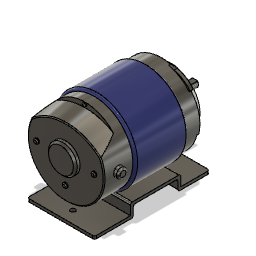
motor (Autodesk Fusion 360 design; units mm, degrees)
Autodesk Fusion 360 part; units mm, degrees
note: some values were not read from the file. Chosen so that the rebuilt part matches the saved one: which face or edge a step refers to. Set by a fixed rule: which sketch regions a step uses.
sketch "Sketch1" plane through (0, 0, 0) normal (0, 0, 1) x (1, 0, 0)
  circle A0 centre (0, 0) radius 42.5
  dimension "d1" = 85
  constraint coincident A0.centre origin
  measures "d1" diameter of A0
extrude "Extrude1" add sketch "Sketch1" along normal mid plane 240
ref_plane "WorkPlane1" through (0, 0, 85) normal (0, 0, 1) x (1, 0, 0)
ref_plane "WorkPlane2" through (0, 0, 95) normal (0, 0, 1) x (1, 0, 0)
sketch "Sketch2" plane through (0, 0, 85) normal (0, 0, 1) x (1, 0, 0)
sketch "Sketch3" plane through (0, 0, 95) normal (0, 0, 1) x (1, 0, 0)
ref_plane "WorkPlane3" through (0, 0, 95) normal (0, 0, 1) x (1, 0, 0)
sketch "Sketch4" plane through (0, 0, 95) normal (0, 0, 1) x (1, 0, 0)
sketch "Sketch5" plane through (0, 0, 95) normal (0, 0, 1) x (1, 0, 0)
sketch "Sketch9" plane through (0, 0, 120) normal (0, 0, 1) x (1, 0, 0)
  circle A0 centre (0, 0) radius 42.5
  arc A1 (41.2919, 10.0612) -> (-41.3271, 9.9158) centre (0.0399, -22.6432) ccw
  arc A2 (41.2919, 10.0612) -> (-41.3271, 9.9158) centre (-0.0158, 8.9798) ccw
  constraint coincident A0 A1.start
  constraint coincident A0 A1.end
extrude "Extrude2" cut sketch "Sketch9" against normal blind 25 contours A0 A1 | A0 A2 picked at (-0.06, 34.0821)
chamfer "Chamfer1" distance 25 distance2 5 1 edges at (-0.0528, 29.9999, 95) measured on face at (15.5458, 27.6646, 103.3333)
sketch "Sketch10" plane through (0, 0, 120) normal (0, 0, 1) x (1, 0, 0)
  arc A0 (41.2919, 10.0612) -> (-41.3271, 9.9158) centre (0.0399, -22.6432) ccw
  arc A1 (-41.3271, 9.9158) -> (41.2919, 10.0612) centre (0, 0) ccw
  circle A2 centre (0, 0) radius 15
  circle A3 centre (0, 0) radius 42.5
  dimension "d12" = 30
  constraint concentric A1 A2
  constraint concentric A2 A3
  measures "d12" diameter of A2
extrude "Extrude3" cut sketch "Sketch10" against normal blind 5
sketch "Sketch11" plane through (0, 0, 0) normal (1, 0, 0) x (0, 0, -1)
sketch "Sketch12" plane through (0, 0, 0) normal (0, 1, 0) x (1, 0, 0)
  line L0 (0, -120) -> (0, 0)
  constraint coincident L0.end origin
sketch "Sketch13" plane through (0, 0, 0) normal (0, 0, 1) x (1, 0, 0)
  circle A0 centre (0, 0) radius 63.2456
  constraint coincident A0.centre origin
extrude "Extrude4" cut sketch "Sketch13" against normal blind 160
sketch "Sketch14" plane through (0, 0, 0) normal (0, 1, 0) x (1, 0, 0)
sketch "Sketch15" plane through (0, 0, 85) normal (0, 0, 1) x (1, 0, 0)
  circle A0 centre (0, 0) radius 40
  circle A1 centre (0, 0) radius 42.5
  circle A2 centre (0, 0) radius 42.5
  arc A3 (36.2233, 22.2288) -> (-36.3014, 22.1011) centre (0, 0) ccw
  dimension "d17" = 80
  constraint coincident A0.centre A1.centre
  constraint concentric A0 A1
  measures "d17" diameter of A0
extrude "Extrude5" cut sketch "Sketch15" along normal blind 90
fillet "Fillet1" radius 2.5 1 edges at (-39.6239, 15.3687, 85)
ref_plane "WorkPlane4" through (0, 0, 30) normal (0, 0, -1) x (-1, 0, 0)
sketch "Sketch16" plane through (0, 0, 30) normal (0, 0, -1) x (1, 0, 0)
  circle A0 centre (0, 0) radius 40
  circle A1 centre (0, 0) radius 42.5
  circle A2 centre (0, 0) radius 42.5
  dimension "d22" = 80
  constraint coincident A0.centre A1.centre
  constraint concentric A0 A1
  measures "d22" diameter of A0
extrude "Extrude6" cut sketch "Sketch16" along normal blind 70
fillet "Fillet2" radius 2 1 edges at (-39.6239, -15.3687, 30)
sketch "Sketch17" plane through (0, 0, 0) normal (0, 0, -1) x (-1, 0, 0)
  circle A0 centre (0, 0) radius 40
  circle A1 centre (0, 0) radius 15
  circle A2 centre (0, 0) radius 15
  dimension "d26" = 30
  constraint concentric A0 A1
  measures "d26" diameter of A1
extrude "Extrude7" cut sketch "Sketch17" against normal blind 5
chamfer "Chamfer2" distance 10 angle 45 1 edges at (-37.2931, -14.4646, 5)
sketch "Sketch18" plane through (0, 0, 0) normal (1, 0, 0) x (0, 0, -1)
sketch "Sketch19" plane through (0, 0, 0) normal (1, 0, 0) x (0, 0, -1)
  line L0 (-115, 15) -> (-115, -15)
  line L1 (-120, 15) -> (-120, -15)
  line L2 (0, -15) -> (0, 15)
  line L3 (-7, 0) -> (-85, 0)
  line L4 (-85, -40) -> (-85, 40)
  line L5 (-15, -40) -> (-15, 40)
  line L6 (-85, 37.8444) -> (-16.9916, 37.8444)
  line L7 (-16.9916, 37.8444) -> (-7, 28)
  line L8 (-7, 28) -> (-7, 0)
  line L9 (-7, 0) -> (-85, 0)
  point P0 (-120, 0)
  constraint coincident L3.end L9.end
  constraint coincident L4 L6.start
  constraint perpendicular L5 L6
  constraint parallel L5 L8
revolve "Revolve1" cut sketch "Sketch19" angle 360 about axis through (0, 0, 7) along (0, 0, 1) contours L3 L4 L5 L6 L7 L9
sketch "Sketch20" plane through (0, 0, 0) normal (0, 0, 1) x (1, 0, 0)
  circle A0 centre (0, 0) radius 4
  constraint coincident A0.centre origin
extrude "Extrude8" cut sketch "Sketch20" along normal blind 57
sketch "Sketch21" plane through (0, 0, 16.9916) normal (0, 0, 1) x (1, 0, 0)
  circle A0 centre (0, 0) radius 37.8444
  circle A1 centre (0, 0) radius 29.3451
  circle A2 centre (0, 0) radius 40
  line L0 (30.8065, 25.5139) -> (23.0524, 18.1583)
  line L1 (6.3754, 28.6442) -> (9.3426, 38.8936)
  arc A3 (30.8065, 25.5139) -> (9.3426, 38.8936) centre (0, 0) ccw
  arc A4 (23.0524, 18.1583) -> (6.3754, 28.6442) centre (-0.1137, -0.1809) ccw
  constraint coincident A2 L0.start
  constraint coincident A1 L0.end
  constraint coincident A1 L1.start
  constraint coincident A2 L1.end
extrude "Extrude10" cut sketch "Sketch21" against normal blind 29 contours A0 A1 L0 L1 | A0 A2 L0 L1 A3 picked at (25.1585, 24.2584)
revolve "Revolve2" cut sketch "Sketch19" angle 360 about axis through (0, 0, 7) along (0, 0, 1)
sketch "Sketch22" plane through (0, 0, 16.9916) normal (0, 0, 1) x (1, 0, 0)
pattern_circular "C-Pattern1" count 4 over 360 about axis through (0, 0, 0) along (0, 0, 1) of "Extrude10"
sketch "Sketch23" plane through (0, 0, 0) normal (1, 0, 0) x (0, 0, -1)
  line L0 (-7, 0) -> (-85, 0)
  line L1 (-16.9916, 28.6442) -> (-16.9916, 18.1583)
  line L2 (-18.3961, 4) -> (-18.3961, 20)
  line L3 (-30, 40) -> (-30, -40)
  line L4 (-30, 40.5) -> (-30, -40.5)
  line L5 (-18.3961, 20) -> (-30, 20)
  line L6 (-30, 27.8576) -> (-65, 27.8576)
  line L7 (-65, 27.8576) -> (-65, 0)
  line L8 (-18.3961, 0) -> (0, 0)
  line L9 (0, 2) -> (0, 4)
  line L10 (0, 0) -> (20, 0)
  line L11 (20, 0) -> (20, 4)
  line L12 (20, 4) -> (-18.3961, 4)
  dimension "d40" = 4
  dimension "d41" = 90
  dimension "d42" = 4
  constraint coincident L0 L8.start
  constraint parallel L1 L2
  constraint coincident L3 L5.end
  constraint coincident L4 L6.start
  constraint perpendicular L4 L6
  constraint coincident L0 L7.end
  constraint perpendicular L0 L7
  constraint coincident L8.end L10.start
  constraint vertical L9
  constraint perpendicular L9 L10
  constraint perpendicular L2 L12
  measures "d40" distance of L8.end L9.end
  measures "d41" angle of L10 L11
  measures "d42" distance of L10.end L11.end
revolve "Revolve3" add sketch "Sketch23" angle 360 about axis through (0, 0, 7) along (0, 0, 1)
fillet "Fillet3" radius 2.5 1 edges at (-18.6465, 7.2323, 18.3961)
sketch "Sketch24" plane through (0, 0, 0) normal (1, 0, 0) x (0, 0, -1)
sketch "Sketch25" plane through (0, 0, -20) normal (0, 0, -1) x (-1, 0, 0)
  circle A0 centre (0, 0) radius 4
  line L0 (-5, 3) -> (5, 3)
  line L1 (5, 3) -> (5, 5.5606)
  line L2 (5, 5.5606) -> (-5, 5.5606)
  line L3 (-5, 5.5606) -> (-5, 3)
  constraint horizontal L0
  constraint perpendicular L0 L1
  constraint perpendicular L1 L2
  constraint perpendicular L0 L3
extrude "Extrude11" cut sketch "Sketch25" against normal blind 12 contours A0 L0 picked at (-0.3801, 3.278)
fillet "Fillet4" radius 0.5 1 edges at (0, -4, -20)
sketch "Sketch26" plane through (0, 0, 0) normal (0, 0, -1) x (-1, 0, 0)
  circle A0 centre (0, 0) radius 4
  circle A1 centre (0, 0) radius 15
  line L0 (-10, 2) -> (-11.7321, 1)
  line L1 (-11.7321, -1) -> (-10, -2)
  line L2 (-10, -2) -> (-8.2679, -1)
  line L3 (-8.2679, -1) -> (-8.2679, 1)
  line L4 (-8.2679, 1) -> (-10, 2)
  line L5 (-11.7321, 1) -> (-11.7321, -1)
  line L6 (10, 2) -> (8.2679, 1)
  line L7 (8.2679, 1) -> (8.2679, -1)
  line L8 (8.2679, -1) -> (10, -2)
  line L9 (10, -2) -> (11.7321, -1)
  line L10 (11.7321, -1) -> (11.7321, 1)
  line L11 (11.7321, 1) -> (10, 2)
  circle A2 centre (10, 0) radius 1.2632
  circle A3 centre (-10, 0) radius 1.2239
  constraint parallel L0 L2
  constraint vertical L3
  constraint parallel L1 L4
  constraint parallel L5 L7
  constraint parallel L6 L9
sketch "Sketch27" plane through (0, 0, 0) normal (0, 0, -1) x (-1, 0, 0)
  line L0 (16, 2.5) -> (16, -2.5)
  line L1 (-16, -2.5) -> (-16, 2.5)
  arc A0 (-10, -2.5) -> (-10, 2.5) centre (-10, 0) ccw
  arc A1 (10, 2.5) -> (10, -2.5) centre (10, 0) ccw
  line L2 (-16, 2.5) -> (-10, 2.5)
  line L3 (10, 2.5) -> (16, 2.5)
  line L4 (16, -2.5) -> (10, -2.5)
  line L5 (-10, -2.5) -> (-16, -2.5)
  constraint horizontal L2
  constraint perpendicular L0 L2
  constraint perpendicular L0 L4
  constraint perpendicular L1 L2
  constraint tangent A0 L4
  constraint tangent A0 L2
  constraint coincident A0.start L4
  constraint tangent A1 L4
  constraint tangent A1 L2
  constraint coincident A1.start L2
  constraint collinear L2 L3
  constraint collinear L4 L5
extrude "Extrude12" cut sketch "Sketch27" against normal blind 2
extrude "Extrude13" add sketch "Sketch26" along normal blind 1 and the other way blind 2 contours L0 L1 L2 L3 L4 L5 | L6 L7 L8 L9 L10 L11
sketch "Sketch28" plane through (0, 0, 0) normal (0, 0, -1) x (-1, 0, 0)
  line L0 (14.7902, -2.5) -> (10, -2.5)
  arc A0 (10, 2.5) -> (10, -2.5) centre (10, 0) ccw
  line L1 (10, 2.5) -> (14.7902, 2.5)
  arc A1 (14.7902, 2.5) -> (-14.7902, 2.5) centre (0, 0) ccw
  line L2 (-14.7902, 2.5) -> (-10, 2.5)
  arc A2 (-10, -2.5) -> (-10, 2.5) centre (-10, 0) ccw
  line L3 (-10, -2.5) -> (-14.7902, -2.5)
  arc A3 (-14.7902, -2.5) -> (14.7902, -2.5) centre (0, 0) ccw
  circle A4 centre (0, 0) radius 4
  circle A5 centre (0, 0) radius 4
  circle A6 centre (0, 0) radius 5
  line L4 (0, -15) -> (0, 15)
  line L5 (0, -40) -> (0, 40)
  constraint coincident A1.centre A3.centre
extrude "Extrude14" cut sketch "Sketch28" against normal blind 2 contours A4 A5 A6 L4 L5 | A4 A5 A6 L4 L5
sketch "Sketch29" plane through (0, 0, 95) normal (0, 0, 1) x (1, 0, 0)
  arc A0 (29.72, 26.7717) -> (-29.814, 26.6669) centre (0, 0) ccw
  arc A1 (29.72, 26.7717) -> (-29.814, 26.6669) centre (0.0399, -22.6432) ccw
  circle A2 centre (0, 37.8444) radius 1.8444
  line L0 (0, -40) -> (0, 40)
  line L1 (0, 37.8444) -> (0, 28)
  point P0 (0, 37.8444)
  constraint coincident P0 A2.centre
extrude "Extrude15" add sketch "Sketch29" along normal blind 2 contours A2 L0 L1 | A2 L0 L1
fillet "Fillet5" radius 1 1 edges at (-1.7196, 37.1774, 97)
sketch "Sketch30" plane through (0, 0, 115) normal (0, 0, 1) x (1, 0, 0)
  arc A0 (-36.2889, 16.8259) -> (36.2295, 16.9536) centre (0, 0) ccw
  arc A1 (36.2295, 16.9536) -> (-36.2889, 16.8259) centre (0.0399, -22.6432) ccw
  circle A2 centre (0, 0) radius 15
  circle A3 centre (30, 0) radius 2.5
  circle A4 centre (-30, 0) radius 2.5
  arc A5 (-29.2745, 6.5579) -> (-23.5295, -18.6108) centre (0, 0) ccw
  circle A6 centre (0, -25) radius 2.5
  line L0 (0, -40) -> (0, 40)
  dimension "d59" = 5
  dimension "d60" = 5
  dimension "d61" = 5
  constraint coincident A4.centre A5
  constraint coincident A6.centre L0
  measures "d59" diameter of A3
  measures "d60" diameter of A4
  measures "d61" diameter of A6
extrude "Extrude16" add sketch "Sketch30" along normal blind 2 contours A6 L0 | A6 L0 | A3 | A4 A5 | A4 A5
chamfer "Chamfer3" distance 1 angle 45 3 edges at (-32.3308, -0.904, 117) (27.6692, -0.904, 117) (-2.3308, -25.904, 117)
chamfer "Chamfer4" distance 2 angle 45 1 edges at (-13.9849, -5.4242, 120)
sketch "Sketch31" plane through (0, 0, 0) normal (0, 0, 1) x (1, 0, 0)
sketch "Sketch32" plane through (0, 0, 0) normal (0, 0, -1) x (-1, 0, 0)
  circle A0 centre (0, 0) radius 5
  line L0 (14.7902, -2.5) -> (10, -2.5)
  arc A1 (10, 2.5) -> (10, -2.5) centre (10, 0) ccw
  line L1 (10, 2.5) -> (14.7902, 2.5)
  arc A2 (14.7902, 2.5) -> (-14.7902, 2.5) centre (0, 0) ccw
  line L2 (-14.7902, 2.5) -> (-10, 2.5)
  arc A3 (-10, -2.5) -> (-10, 2.5) centre (-10, 0) ccw
  line L3 (-10, -2.5) -> (-14.7902, -2.5)
  arc A4 (-14.7902, -2.5) -> (14.7902, -2.5) centre (0, 0) ccw
  line L4 (0, -40) -> (0, 40)
  line L5 (0, 0) -> (0, -75)
  line L6 (0, -75) -> (45, -75)
  line L7 (45, -75) -> (45, -40)
  circle A5 centre (0, 0) radius 42.5
  line L8 (0, -75) -> (-45, -75)
  line L9 (-45, -75) -> (-45, -40)
  arc A6 (-14.3614, -40) -> (14.3614, -40) centre (0, 0) ccw
  line L10 (-45, -40) -> (-14.3614, -40)
  line L11 (14.3614, -40) -> (45, -40)
  constraint coincident A0.centre A2.centre
  constraint parallel L4 L5
  constraint perpendicular L5 L6
  constraint perpendicular L6 L7
  constraint perpendicular L5 L8
  constraint perpendicular L8 L9
  constraint perpendicular L7 L10
  constraint coincident A6.end L10
  constraint coincident A5 A6.end
  constraint coincident A5 A6.start
  constraint collinear L10 L11
extrude "Extrude17" add sketch "Sketch32" against normal blind 120 contours L5 L6 L7 A5 A6 L11 | L5 A5 L8 L9 A6 L10
sketch "Sketch33" plane through (-45, 0, 0) normal (-1, 0, 0) x (0, 0, 1)
  line L0 (0, -40) -> (0, -75)
  line L1 (0, -75) -> (120, -75)
  line L2 (120, -75) -> (120, -40)
  line L3 (120, -40) -> (0, -40)
  line L4 (30, -40) -> (-10, -40)
  line L5 (-10, -40) -> (-10, -72)
  line L6 (-10, -72) -> (30, -72)
  line L7 (30, -72) -> (30, -40)
  line L8 (82.5, -40) -> (82.5, -72)
  line L9 (82.5, -72) -> (127.3639, -72)
  line L10 (127.3639, -72) -> (125, -40)
  line L11 (125, -40) -> (82.5, -40)
  point P0 (82.5, -40)
  point P1 (82.5, -40)
  dimension "d70" = 90
  dimension "d71" = 32
  constraint coincident L3 L4.start
  constraint perpendicular L0 L4
  constraint perpendicular L0 L6
  constraint perpendicular L4 L7
  constraint coincident P1 P0
  constraint perpendicular L3 L8
  constraint perpendicular L2 L9
  constraint perpendicular L8 L11
  measures "d70" angle of L4 L5
  measures "d71" distance of L4.end L5.end
extrude "Extrude18" cut sketch "Sketch33" against normal blind 320 contours L0 L3 L4 L6 L7 | L0 L4 L5 L6 | L2 L3 L8 L9 L11 | L2 L9 L10 L11
sketch "Sketch34" plane through (-45, 0, 0) normal (-1, 0, 0) x (0, 0, 1)
  line L0 (30, -72) -> (0, -72)
  line L1 (0, -72) -> (0, -75)
  line L2 (0, -75) -> (120, -75)
  line L3 (120, -75) -> (120, -72)
  line L4 (120, -72) -> (82.5, -72)
  line L5 (82.5, -40) -> (30, -40)
  line L6 (33, -43) -> (33, -72)
  line L7 (79.5, -72) -> (79.5, -43)
  line L8 (79.5, -43) -> (33, -43)
  line L9 (33, -72) -> (33, -81.992)
  line L10 (79.5, -72) -> (79.5, -81.8501)
  line L11 (79.5, -81.8501) -> (35.0278, -81.992)
  line L12 (35.0278, -81.992) -> (33, -81.992)
  constraint parallel L5 L8
  constraint perpendicular L2 L9
  constraint perpendicular L2 L10
  constraint perpendicular L9 L12
extrude "Extrude19" cut sketch "Sketch34" against normal blind 120
sketch "Sketch35" plane through (0, 0, 30) normal (0, 0, -1) x (-1, 0, 0)
  arc A0 (-14.3614, -40) -> (14.3614, -40) centre (0, 0) ccw
  line L0 (-14.3614, -40) -> (-45, -40)
  line L1 (-45, -40) -> (-45, -72)
  line L2 (-45, -72) -> (45, -72)
  line L3 (45, -72) -> (45, -40)
  line L4 (45, -40) -> (14.3614, -40)
  line L5 (-35, -40) -> (-35, -87.1803)
  line L6 (-35, -87.1803) -> (-60.0488, -77.3043)
  line L7 (-60.0488, -77.3043) -> (-58.0333, -25.1025)
  line L8 (-58.0333, -25.1025) -> (-35, -31.9553)
  line L9 (-35, -31.9553) -> (-35, -40)
  line L10 (35, -85) -> (35, -31.9553)
  line L11 (35, -31.9553) -> (53.2229, -31.9553)
  line L12 (53.2229, -31.9553) -> (50, -85)
  line L13 (50, -85) -> (35, -85)
  constraint coincident L0 L5.start
  constraint perpendicular L2 L5
  constraint perpendicular L0 L9
  constraint perpendicular L2 L10
  constraint perpendicular L10 L11
  constraint perpendicular L10 L13
extrude "Extrude20" cut sketch "Sketch35" along normal mid plane 270 contours L0 L1 L2 L5 | L0 L1 L2 L5 L6 L7 L8 L9 | L2 L3 L4 L10 L11 L12 L13 | L2 L3 L4 L10
fillet "Fillet6" radius 2 1 edges at (0, -72, 30)
fillet "Fillet7" radius 2 5 edges at (24.6807, -40, 30) (-24.6807, -40, 30) (-24.6807, -40, 82.5) (24.6807, -40, 82.5) (0, -72, 82.5)
fillet "Fillet8" radius 2 4 edges at (0, -75, 33) (0, -43, 33) (0, -43, 79.5) (0, -75, 79.5)
sketch "Sketch36" plane through (0, -72, 0) normal (0, 1, 0) x (-1, 0, 0)
  line L0 (35, 28) -> (-35, 28)
  line L1 (-35, 28) -> (-35, 0)
  line L2 (-35, 0) -> (35, 0)
  line L3 (35, 0) -> (35, 28)
  line L4 (0, 16.9916) -> (0, 7)
  line L5 (0, 11.9958) -> (0, 96.9958)
  line L6 (-25, 14.9958) -> (25, 14.9958)
  line L7 (25, 14.9958) -> (25, 8.9958)
  line L8 (25, 8.9958) -> (-25, 8.9958)
  line L9 (-25, 8.9958) -> (-25, 14.9958)
  line L10 (-25, 14.9958) -> (25, 8.9958) construction
  line L11 (25, 14.9958) -> (-25, 8.9958) construction
  line L12 (-25, 99.9958) -> (25, 99.9958)
  line L13 (25, 99.9958) -> (25, 93.9958)
  line L14 (25, 93.9958) -> (-25, 93.9958)
  line L15 (-25, 93.9958) -> (-25, 99.9958)
  line L16 (-25, 99.9958) -> (25, 93.9958) construction
  line L17 (25, 99.9958) -> (-25, 93.9958) construction
  point P0 (0, 11.9958)
  point P1 (0, 96.9958)
  dimension "d82" = 85
  dimension "d83" = 50
  dimension "d84" = 6
  dimension "d85" = 50
  dimension "d86" = 6
  constraint midpoint L4 P0
  constraint perpendicular L0 L5
  constraint perpendicular L6 L7
  constraint parallel L6 L8
  constraint parallel L7 L9
  constraint horizontal L6
  constraint coincident L10 P0
  constraint coincident L11 P0
  constraint coincident P0 L5.start
  constraint perpendicular L12 L13
  constraint parallel L12 L14
  constraint parallel L13 L15
  constraint horizontal L12
  constraint coincident L16 P1
  constraint coincident L17 P1
  constraint coincident P1 L5.end
  measures "d82" distance of P0 P1
  measures "d83" distance of L7.end L8.end
  measures "d84" distance of L6.end L7.end
  measures "d85" distance of L13.end L14.end
  measures "d86" distance of L12.end L13.end
extrude "Extrude21" cut sketch "Sketch36" against normal blind 20 contours L4 L5 L6 L7 L8 | L4 L5 L6 L8 L9 | L12 L13 L14 L15
fillet "Fillet9" radius 2 8 edges at (35, -73.5, 0) (-35, -73.5, 0) (25, -73.5, 14.9958) (25, -73.5, 8.9958) (-25, -73.5, 8.9958) (35, -73.5, 120) (-25, -73.5, 14.9958) (-35, -73.5, 120)
fillet "Fillet10" radius 2 4 edges at (25, -73.5, 93.9958) (25, -73.5, 99.9958) (-25, -73.5, 99.9958) (-25, -73.5, 93.9958)
fillet "Fillet11" radius 1 2 edges at (0, 15, 0) (0, -15, 0)
sketch "Sketch37" plane through (0, 0, 16.9916) normal (0, 0, 1) x (1, 0, 0)
sketch "Sketch38" plane through (0, 0, 0) normal (1, 0, 0) x (0, 0, -1)
  circle A0 centre (-100, 0) radius 5
  dimension "d92" = 10
  measures "d92" diameter of A0
sketch "Sketch39" plane through (0, 0, 0) normal (1, 0, 0) x (0, 0, -1)
  circle A0 centre (-100, 0) radius 5
  circle A1 centre (-100, 0) radius 5
  point P0 (-100, 0)
  constraint coincident P0 A0.centre
extrude "Extrude22" add sketch "Sketch39" along normal mid plane 100
fillet "Fillet12" radius 5 2 edges at (-50, 1.8081, 104.6616) (50, -1.8081, 104.6616)
sketch "Sketch40" plane through (0, 0, 0) normal (0, 1, 0) x (1, 0, 0)
  line L0 (-45, -95) -> (-45, -105)
  line L1 (-45, -109.0529) -> (-45, -86.6148)
  line L2 (-45, -86.6148) -> (-63.8915, -86.6148)
  line L3 (-63.8915, -86.6148) -> (-65.793, -112.4757)
  line L4 (-65.793, -112.4757) -> (-45, -109.0529)
  line L5 (44.686, -112.4757) -> (45, -85)
  line L6 (45, -85) -> (57.046, -98.7378)
  line L7 (57.046, -98.7378) -> (44.686, -112.4757)
  constraint parallel L0 L1
  constraint perpendicular L0 L2
extrude "Extrude23" cut sketch "Sketch40" along normal mid plane 130
fillet "Fillet13" radius 2 1 edges at (-45, 1.8081, 104.6616)
fillet "Fillet14" radius 2 1 edges at (44.7714, 0, 105)
sketch "Sketch41" plane through (0, 0, 0) normal (1, 0, 0) x (0, 0, -1)
fillet "Fillet15" radius 1 2 edges at (0.0704, -39.9999, 115) (-0.0546, 30.9999, 115)
sketch "Sketch42" plane through (0, 0, 0) normal (1, 0, 0) x (0, 0, -1)
  line L0 (20, -54.5) -> (-150, -54.5)
  line L1 (20, -54.5) -> (15, -85)
  line L2 (15, -85) -> (-142.3105, -85)
  line L3 (-142.3105, -85) -> (-150, -54.5)
  point P0 (20, 0)
  dimension "d101" = 54.5
  constraint parallel L0 L2
  measures "d101" distance of P0 L0.start
extrude "Extrude24" cut sketch "Sketch42" along normal mid plane 130
sketch "Sketch43" plane through (0, 0, 0) normal (1, 0, 0) x (0, 0, -1)
  line L0 (20, 0) -> (19.5255, -54.4979)
  line L1 (-33, -54.5) -> (0, -54.5)
  line L2 (0, -54.5) -> (0, -51.5)
  line L3 (-33, -54.5) -> (-33, -45)
  line L4 (0, -51.5) -> (-33, -51.5)
  line L5 (-33, -54.5) -> (-33, -51.5)
  line L6 (-120, -75) -> (-120, -40)
  line L7 (-79.5, -54.5) -> (-120, -54.5)
  line L8 (-120, -54.5) -> (-120, -51.5)
  line L9 (-79.5, -45) -> (-79.5, -54.5)
  line L10 (-120, -51.5) -> (-79.5, -51.5)
  line L11 (-79.5, -51.5) -> (-79.5, -54.5)
  line L12 (0, -51.5) -> (0, -54.5)
  line L13 (-120, -54.5) -> (-120, -51.5)
  point P0 (20, 0)
  point P1 (-33, -54.5)
  point P2 (-79.5, -54.5)
  point P3 (-79.5, -54.5)
  dimension "d104" = 54.5
  dimension "d105" = 3
  constraint coincident P0 L0.start
  constraint coincident P1 L1.start
  constraint coincident L3 L4.end
  constraint perpendicular L2 L4
  constraint perpendicular L4 L5
  constraint coincident P3 P2
  constraint coincident L6 L7.end
  constraint perpendicular L3 L7
  constraint coincident L6 L8.end
  constraint coincident L9 L10.end
  constraint perpendicular L8 L10
  measures "d104" distance of P0 L0.end
  measures "d105" distance of L1.end L2.end
extrude "Extrude25" add sketch "Sketch43" along normal mid plane 70
sketch "Sketch44" plane through (0, -54.5, 0) normal (0, -1, 0) x (1, 0, 0)
  line L0 (35, 0) -> (35, 33)
  line L1 (35, 33) -> (-35, 33)
  line L2 (-35, 33) -> (-35, 0)
  line L3 (-35, 0) -> (35, 0)
extrude "Extrude26" cut sketch "Sketch36" along normal blind 30 contours L4 L5 L6 L7 L8 | L4 L5 L6 L8 L9 | L12 L13 L14 L15
fillet "Fillet16" radius 2 6 edges at (35, -53, 0) (-35, -53, 0) (-35, -53, 120) (35, -53, 120) (0, -54.5, 33) (0, -54.5, 79.5)
move_face "OffsetFaces1" offset 14 1 faces at (-8.3333, -53.5, 93.9958)
move_face "OffsetFaces2" offset 8 1 faces at (8.3333, -53.5, 14.9958)
sketch "Sketch45" plane through (0, -51.5, 0) normal (0, 1, 0) x (-1, 0, 0)
  arc A0 (33, 0) -> (35, 2) centre (33, 2) ccw
  line L0 (35, 2) -> (35, 30)
  line L1 (35, 30) -> (-35, 30)
  line L2 (-35, 30) -> (-35, 2)
  arc A1 (-35, 2) -> (-33, 0) centre (-33, 2) ccw
  line L3 (-33, 0) -> (33, 0)
sketch "Sketch46" plane through (0, -54.5, 0) normal (0, -1, 0) x (1, 0, 0)
  line L0 (-35, 81.5) -> (35, 81.5)
  line L1 (35, 81.5) -> (35, 118)
  arc A0 (35, 118) -> (33, 120) centre (33, 118) ccw
  line L2 (33, 120) -> (-33, 120)
  arc A1 (-33, 120) -> (-35, 118) centre (-33, 118) ccw
  line L3 (-35, 118) -> (-35, 81.5)
  line L4 (0, 110) -> (0, 107.5)
  circle A2 centre (0, 107.5) radius 2.5
  line L5 (0, 120) -> (0, 0)
  line L6 (0, 107.5) -> (0, 22.5)
  circle A3 centre (0, 22.5) radius 2.5
  point P0 (0, 120)
  dimension "d113" = 12.5
  dimension "d114" = 85
  dimension "d115" = 5
  constraint coincident L4.end A2.centre
  constraint coincident A2 L4.start
  constraint coincident L6.end A3.centre
  measures "d113" distance of P0 L4.end
  measures "d114" distance of L4.end L6.end
  measures "d115" diameter of A3
extrude "Extrude27" cut sketch "Sketch46" against normal blind 6 contours L4 A2 L5 L6 | L4 A2 L5 L6 | L5 L6 A3 | L5 L6 A3
sketch "Sketch47" plane through (0, -54.5, 0) normal (0, -1, 0) x (1, 0, 0)
  circle A0 centre (0, 107.5) radius 2.5
  line L0 (-35, 81.5) -> (35, 81.5)
  line L1 (35, 81.5) -> (35, 118)
  arc A1 (35, 118) -> (33, 120) centre (33, 118) ccw
  line L2 (33, 120) -> (-33, 120)
  arc A2 (-33, 120) -> (-35, 118) centre (-33, 118) ccw
  line L3 (-35, 118) -> (-35, 81.5)
extrude "Extrude9" [suppressed]
